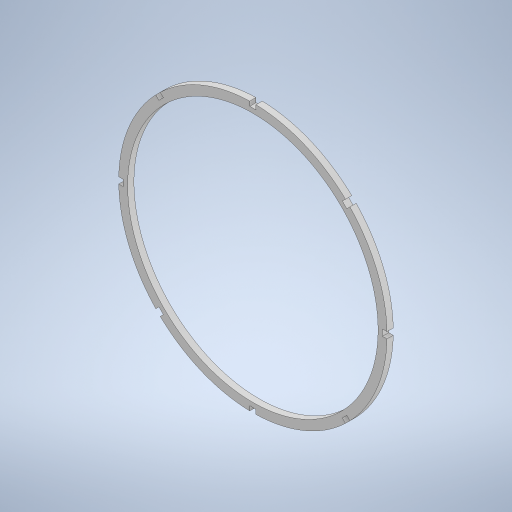
# Autodesk Inventor part: Sirsi obroc
Saved by Autodesk Inventor 2023 (Build 270158000, 158)
## iProperties
Created: 2022-12-16
Part Number: Sirsi obroc
Material: Generic
Document SubType Name: Modeling
Designer: David Zindović
Density: 1 g/cm^3
Appearance: Default
Author: David Zindović
Autodesk Inventor part; units mm, degrees
ref_plane "YZ Plane" through (0, 0, 0) normal (1, 0, 0) x (0, 1, 0)
ref_plane "XZ Plane" through (0, 0, 0) normal (0, 1, 0) x (-1, 0, 0)
ref_plane "XY Plane" through (0, 0, 0) normal (0, 0, 1) x (1, 0, 0)
sketch "Sketch1" plane through (0, 0, 0) normal (0, 0, 1) x (1, 0, 0)
  circle A0 centre (0, 0) radius 70
  circle A1 centre (0, 0) radius 75
  line L0 (72.5, 1.75) -> (75, 1.75)
  line L1 (75, 1.75) -> (75, 0)
  line L2 (75, 0) -> (72.5, 0)
  line L3 (72.5, 0) -> (72.5, 1.75)
  line L4 (70, 0) -> (75, 0)
  line L5 (72.5, -1.75) -> (75, -1.75)
  line L6 (75, -1.75) -> (75, 0)
  line L7 (72.5, 0) -> (72.5, -1.75)
  line L8 (51.2652, 51.2652) -> (50.0278, 52.5027)
  line L9 (50.0278, 52.5027) -> (51.7956, 54.2704)
  line L10 (52.5027, 50.0278) -> (54.2704, 51.7956)
  line L11 (51.2652, 51.2652) -> (52.5027, 50.0278)
  line L12 (54.2704, 51.7956) -> (53.033, 53.033)
  line L13 (51.7956, 54.2704) -> (53.033, 53.033)
  line L14 (0, 72.5) -> (-1.75, 72.5)
  line L15 (-1.75, 72.5) -> (-1.75, 75)
  line L16 (1.75, 72.5) -> (1.75, 75)
  line L17 (0, 72.5) -> (1.75, 72.5)
  line L18 (1.75, 75) -> (0, 75)
  line L19 (-1.75, 75) -> (0, 75)
  line L20 (-51.2652, 51.2652) -> (-52.5027, 50.0278)
  line L21 (-52.5027, 50.0278) -> (-54.2704, 51.7956)
  line L22 (-50.0278, 52.5027) -> (-51.7956, 54.2704)
  line L23 (-51.2652, 51.2652) -> (-50.0278, 52.5027)
  line L24 (-51.7956, 54.2704) -> (-53.033, 53.033)
  line L25 (-54.2704, 51.7956) -> (-53.033, 53.033)
  line L26 (-72.5, 0) -> (-72.5, -1.75)
  line L27 (-72.5, -1.75) -> (-75, -1.75)
  line L28 (-72.5, 1.75) -> (-75, 1.75)
  line L29 (-72.5, 0) -> (-72.5, 1.75)
  line L30 (-75, 1.75) -> (-75, 0)
  line L31 (-75, -1.75) -> (-75, 0)
  line L32 (-51.2652, -51.2652) -> (-50.0278, -52.5027)
  line L33 (-50.0278, -52.5027) -> (-51.7956, -54.2704)
  line L34 (-52.5027, -50.0278) -> (-54.2704, -51.7956)
  line L35 (-51.2652, -51.2652) -> (-52.5027, -50.0278)
  line L36 (-54.2704, -51.7956) -> (-53.033, -53.033)
  line L37 (-51.7956, -54.2704) -> (-53.033, -53.033)
  line L38 (0, -72.5) -> (1.75, -72.5)
  line L39 (1.75, -72.5) -> (1.75, -75)
  line L40 (-1.75, -72.5) -> (-1.75, -75)
  line L41 (0, -72.5) -> (-1.75, -72.5)
  line L42 (-1.75, -75) -> (0, -75)
  line L43 (1.75, -75) -> (0, -75)
  line L44 (51.2652, -51.2652) -> (52.5027, -50.0278)
  line L45 (52.5027, -50.0278) -> (54.2704, -51.7956)
  line L46 (50.0278, -52.5027) -> (51.7956, -54.2704)
  line L47 (51.2652, -51.2652) -> (50.0278, -52.5027)
  line L48 (51.7956, -54.2704) -> (53.033, -53.033)
  line L49 (54.2704, -51.7956) -> (53.033, -53.033)
  point P0 (74.9796, 1.75)
  point P1 (54.256, 51.7811)
  point P2 (51.7811, 54.256)
  point P3 (1.75, 74.9796)
  point P4 (-1.75, 74.9796)
  point P5 (-51.7811, 54.256)
  point P6 (-54.256, 51.7811)
  point P7 (-74.9796, 1.75)
  point P8 (-74.9796, -1.75)
  point P9 (-54.256, -51.7811)
  point P10 (-51.7811, -54.256)
  point P11 (-1.75, -74.9796)
  point P12 (1.75, -74.9796)
  point P13 (51.7811, -54.256)
  point P14 (54.256, -51.7811)
  point P15 (74.9796, -1.75)
  dimension "d0" = 140
  dimension "d1" = 5
  dimension "d2" = 1.75
  dimension "d5" = 360
  constraints: 100 end point, 2 horizontal, 2 parallel, 2 symmetric about line, 1 coincident, 1 horizontal alignment, 1 midpoint, 1 perpendicular, 1 vertical alignment, 102 other
  measures "d2" distance of L2.end L0.start
extrude "Extrusion1" add sketch "Sketch1" along normal mid plane 3.5 contours L7 L5 A1 L45 L44 L47 L46 L39 L38 L41 L40 L33 L32 L35 L34 L27 L26 L29 L28 L21 L20 L23 L22 L15 L14 L17 L16 L9 L8 L11 L10 L0 L3
body "Solid1"
